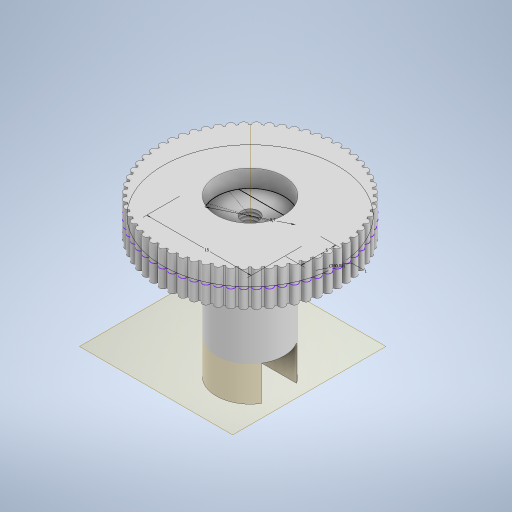
# Autodesk Inventor part: Justage_Knopf
Saved by Autodesk Inventor 2024 (Build 280153000, 153)
## iProperties
Created: 2024-03-07
Part Number: Justage_Knopf
Material: Generisch
Document SubType Name: Modeling
Designer: s1alknau
Density: 1 g/cm^3
Appearance: Vorgabe
Author: s1alknau
Autodesk Inventor part; units mm, degrees
ref_plane "YZ Plane" through (0, 0, 0) normal (1, 0, 0) x (0, 1, 0)
ref_plane "XZ Plane" through (0, 0, 0) normal (0, 1, 0) x (-1, 0, 0)
ref_plane "XY Plane" through (0, 0, 0) normal (0, 0, 1) x (1, 0, 0)
sketch "Skizze1" plane through (0, 0, 0) normal (0, 0, 1) x (1, 0, 0)
  circle A0 centre (0, 0) radius 4.85
  arc A1 (12.49, -0.4999) -> (12.49, 0.4999) centre (12.5, 0) ccw
  arc A2 (12.4738, 0.8084) -> (12.3693, 1.8027) centre (12.4315, 1.3066) ccw
  arc A3 (12.321, 2.1078) -> (12.1131, 3.0858) centre (12.2268, 2.5989) ccw
  arc A4 (12.0332, 3.3842) -> (11.7242, 4.3351) centre (11.8882, 3.8627) ccw
  arc A5 (11.6135, 4.6235) -> (11.2069, 5.5368) centre (11.4193, 5.0842) ccw
  arc A6 (11.0666, 5.8121) -> (10.5667, 6.6779) centre (10.8253, 6.25) ccw
  arc A7 (10.3985, 6.937) -> (9.8108, 7.7459) centre (10.1127, 7.3473) ccw
  arc A8 (9.6164, 7.9859) -> (8.9474, 8.7289) centre (9.2893, 8.3641) ccw
  arc A9 (8.7289, 8.9474) -> (7.9859, 9.6164) centre (8.3641, 9.2893) ccw
  arc A10 (7.7459, 9.8108) -> (6.937, 10.3985) centre (7.3473, 10.1127) ccw
  arc A11 (6.6779, 10.5667) -> (5.8121, 11.0666) centre (6.25, 10.8253) ccw
  arc A12 (5.5368, 11.2069) -> (4.6235, 11.6135) centre (5.0842, 11.4193) ccw
  arc A13 (4.3351, 11.7242) -> (3.3842, 12.0332) centre (3.8627, 11.8882) ccw
  arc A14 (3.0858, 12.1131) -> (2.1078, 12.321) centre (2.5989, 12.2268) ccw
  arc A15 (1.8027, 12.3693) -> (0.8084, 12.4738) centre (1.3066, 12.4315) ccw
  arc A16 (0.4999, 12.49) -> (-0.4999, 12.49) centre (0, 12.5) ccw
  arc A17 (-0.8084, 12.4738) -> (-1.8027, 12.3693) centre (-1.3066, 12.4315) ccw
  arc A18 (-2.1078, 12.321) -> (-3.0858, 12.1131) centre (-2.5989, 12.2268) ccw
  arc A19 (-3.3842, 12.0332) -> (-4.3351, 11.7242) centre (-3.8627, 11.8882) ccw
  arc A20 (-4.6235, 11.6135) -> (-5.5368, 11.2069) centre (-5.0842, 11.4193) ccw
  arc A21 (-5.8121, 11.0666) -> (-6.6779, 10.5667) centre (-6.25, 10.8253) ccw
  arc A22 (-6.937, 10.3985) -> (-7.7459, 9.8108) centre (-7.3473, 10.1127) ccw
  arc A23 (-7.9859, 9.6164) -> (-8.7289, 8.9474) centre (-8.3641, 9.2893) ccw
  arc A24 (-8.9474, 8.7289) -> (-9.6164, 7.9859) centre (-9.2893, 8.3641) ccw
  arc A25 (-9.8108, 7.7459) -> (-10.3985, 6.937) centre (-10.1127, 7.3473) ccw
  arc A26 (-10.5667, 6.6779) -> (-11.0666, 5.8121) centre (-10.8253, 6.25) ccw
  arc A27 (-11.2069, 5.5368) -> (-11.6135, 4.6235) centre (-11.4193, 5.0842) ccw
  arc A28 (-11.7242, 4.3351) -> (-12.0332, 3.3842) centre (-11.8882, 3.8627) ccw
  arc A29 (-12.1131, 3.0858) -> (-12.321, 2.1078) centre (-12.2268, 2.5989) ccw
  arc A30 (-12.3693, 1.8027) -> (-12.4738, 0.8084) centre (-12.4315, 1.3066) ccw
  arc A31 (-12.49, 0.4999) -> (-12.49, -0.4999) centre (-12.5, 0) ccw
  arc A32 (-12.4738, -0.8084) -> (-12.3693, -1.8027) centre (-12.4315, -1.3066) ccw
  arc A33 (-12.321, -2.1078) -> (-12.1131, -3.0858) centre (-12.2268, -2.5989) ccw
  arc A34 (-12.0332, -3.3842) -> (-11.7242, -4.3351) centre (-11.8882, -3.8627) ccw
  arc A35 (-11.6135, -4.6235) -> (-11.2069, -5.5368) centre (-11.4193, -5.0842) ccw
  arc A36 (-11.0666, -5.8121) -> (-10.5667, -6.6779) centre (-10.8253, -6.25) ccw
  arc A37 (-10.3985, -6.937) -> (-9.8108, -7.7459) centre (-10.1127, -7.3473) ccw
  arc A38 (-9.6164, -7.9859) -> (-8.9474, -8.7289) centre (-9.2893, -8.3641) ccw
  arc A39 (-8.7289, -8.9474) -> (-7.9859, -9.6164) centre (-8.3641, -9.2893) ccw
  arc A40 (-7.7459, -9.8108) -> (-6.937, -10.3985) centre (-7.3473, -10.1127) ccw
  arc A41 (-6.6779, -10.5667) -> (-5.8121, -11.0666) centre (-6.25, -10.8253) ccw
  arc A42 (-5.5368, -11.2069) -> (-4.6235, -11.6135) centre (-5.0842, -11.4193) ccw
  arc A43 (-4.3351, -11.7242) -> (-3.3842, -12.0332) centre (-3.8627, -11.8882) ccw
  arc A44 (-3.0858, -12.1131) -> (-2.1078, -12.321) centre (-2.5989, -12.2268) ccw
  arc A45 (-1.8027, -12.3693) -> (-0.8084, -12.4738) centre (-1.3066, -12.4315) ccw
  arc A46 (-0.4999, -12.49) -> (0.4999, -12.49) centre (0, -12.5) ccw
  arc A47 (0.8084, -12.4738) -> (1.8027, -12.3693) centre (1.3066, -12.4315) ccw
  arc A48 (2.1078, -12.321) -> (3.0858, -12.1131) centre (2.5989, -12.2268) ccw
  arc A49 (3.3842, -12.0332) -> (4.3351, -11.7242) centre (3.8627, -11.8882) ccw
  arc A50 (4.6235, -11.6135) -> (5.5368, -11.2069) centre (5.0842, -11.4193) ccw
  arc A51 (5.8121, -11.0666) -> (6.6779, -10.5667) centre (6.25, -10.8253) ccw
  arc A52 (6.937, -10.3985) -> (7.7459, -9.8108) centre (7.3473, -10.1127) ccw
  arc A53 (7.9859, -9.6164) -> (8.7289, -8.9474) centre (8.3641, -9.2893) ccw
  arc A54 (8.9474, -8.7289) -> (9.6164, -7.9859) centre (9.2893, -8.3641) ccw
  arc A55 (9.8108, -7.7459) -> (10.3985, -6.937) centre (10.1127, -7.3473) ccw
  arc A56 (10.5667, -6.6779) -> (11.0666, -5.8121) centre (10.8253, -6.25) ccw
  arc A57 (11.2069, -5.5368) -> (11.6135, -4.6235) centre (11.4193, -5.0842) ccw
  arc A58 (11.7242, -4.3351) -> (12.0332, -3.3842) centre (11.8882, -3.8627) ccw
  arc A59 (12.1131, -3.0858) -> (12.321, -2.1078) centre (12.2268, -2.5989) ccw
  arc A60 (12.3693, -1.8027) -> (12.4738, -0.8084) centre (12.4315, -1.3066) ccw
  arc A61 (12.4738, -0.8084) -> (12.49, -0.4999) centre (0, 0) ccw
  arc A62 (12.321, -2.1078) -> (12.3693, -1.8027) centre (0, 0) ccw
  arc A63 (12.0332, -3.3842) -> (12.1131, -3.0858) centre (0, 0) ccw
  arc A64 (11.6135, -4.6235) -> (11.7242, -4.3351) centre (0, 0) ccw
  arc A65 (11.0666, -5.8121) -> (11.2069, -5.5368) centre (0, 0) ccw
  arc A66 (10.3985, -6.937) -> (10.5667, -6.6779) centre (0, 0) ccw
  arc A67 (9.6164, -7.9859) -> (9.8108, -7.7459) centre (0, 0) ccw
  arc A68 (8.7289, -8.9474) -> (8.9474, -8.7289) centre (0, 0) ccw
  arc A69 (7.7459, -9.8108) -> (7.9859, -9.6164) centre (0, 0) ccw
  arc A70 (6.6779, -10.5667) -> (6.937, -10.3985) centre (0, 0) ccw
  arc A71 (5.5368, -11.2069) -> (5.8121, -11.0666) centre (0, 0) ccw
  arc A72 (4.3351, -11.7242) -> (4.6235, -11.6135) centre (0, 0) ccw
  arc A73 (3.0858, -12.1131) -> (3.3842, -12.0332) centre (0, 0) ccw
  arc A74 (1.8027, -12.3693) -> (2.1078, -12.321) centre (0, 0) ccw
  arc A75 (0.4999, -12.49) -> (0.8084, -12.4738) centre (0, 0) ccw
  arc A76 (-0.8084, -12.4738) -> (-0.4999, -12.49) centre (0, 0) ccw
  arc A77 (-2.1078, -12.321) -> (-1.8027, -12.3693) centre (0, 0) ccw
  arc A78 (-3.3842, -12.0332) -> (-3.0858, -12.1131) centre (0, 0) ccw
  arc A79 (-4.6235, -11.6135) -> (-4.3351, -11.7242) centre (0, 0) ccw
  arc A80 (-5.8121, -11.0666) -> (-5.5368, -11.2069) centre (0, 0) ccw
  arc A81 (-6.937, -10.3985) -> (-6.6779, -10.5667) centre (0, 0) ccw
  arc A82 (-7.9859, -9.6164) -> (-7.7459, -9.8108) centre (0, 0) ccw
  arc A83 (-8.9474, -8.7289) -> (-8.7289, -8.9474) centre (0, 0) ccw
  arc A84 (-9.8108, -7.7459) -> (-9.6164, -7.9859) centre (0, 0) ccw
  arc A85 (-10.5667, -6.6779) -> (-10.3985, -6.937) centre (0, 0) ccw
  arc A86 (-11.2069, -5.5368) -> (-11.0666, -5.8121) centre (0, 0) ccw
  arc A87 (-11.7242, -4.3351) -> (-11.6135, -4.6235) centre (0, 0) ccw
  arc A88 (-12.1131, -3.0858) -> (-12.0332, -3.3842) centre (0, 0) ccw
  arc A89 (-12.3693, -1.8027) -> (-12.321, -2.1078) centre (0, 0) ccw
  arc A90 (-12.49, -0.4999) -> (-12.4738, -0.8084) centre (0, 0) ccw
  arc A91 (-12.4738, 0.8084) -> (-12.49, 0.4999) centre (0, 0) ccw
  arc A92 (-12.321, 2.1078) -> (-12.3693, 1.8027) centre (0, 0) ccw
  arc A93 (-12.0332, 3.3842) -> (-12.1131, 3.0858) centre (0, 0) ccw
  arc A94 (-11.6135, 4.6235) -> (-11.7242, 4.3351) centre (0, 0) ccw
  arc A95 (-11.0666, 5.8121) -> (-11.2069, 5.5368) centre (0, 0) ccw
  arc A96 (-10.3985, 6.937) -> (-10.5667, 6.6779) centre (0, 0) ccw
  arc A97 (-9.6164, 7.9859) -> (-9.8108, 7.7459) centre (0, 0) ccw
  arc A98 (-8.7289, 8.9474) -> (-8.9474, 8.7289) centre (0, 0) ccw
  arc A99 (-7.7459, 9.8108) -> (-7.9859, 9.6164) centre (0, 0) ccw
  arc A100 (-6.6779, 10.5667) -> (-6.937, 10.3985) centre (0, 0) ccw
  arc A101 (-5.5368, 11.2069) -> (-5.8121, 11.0666) centre (0, 0) ccw
  arc A102 (-4.3351, 11.7242) -> (-4.6235, 11.6135) centre (0, 0) ccw
  arc A103 (-3.0858, 12.1131) -> (-3.3842, 12.0332) centre (0, 0) ccw
  arc A104 (-1.8027, 12.3693) -> (-2.1078, 12.321) centre (0, 0) ccw
  arc A105 (-0.4999, 12.49) -> (-0.8084, 12.4738) centre (0, 0) ccw
  arc A106 (0.8084, 12.4738) -> (0.4999, 12.49) centre (0, 0) ccw
  arc A107 (2.1078, 12.321) -> (1.8027, 12.3693) centre (0, 0) ccw
  arc A108 (3.3842, 12.0332) -> (3.0858, 12.1131) centre (0, 0) ccw
  arc A109 (4.6235, 11.6135) -> (4.3351, 11.7242) centre (0, 0) ccw
  arc A110 (5.8121, 11.0666) -> (5.5368, 11.2069) centre (0, 0) ccw
  arc A111 (6.937, 10.3985) -> (6.6779, 10.5667) centre (0, 0) ccw
  arc A112 (7.9859, 9.6164) -> (7.7459, 9.8108) centre (0, 0) ccw
  arc A113 (8.9474, 8.7289) -> (8.7289, 8.9474) centre (0, 0) ccw
  arc A114 (9.8108, 7.7459) -> (9.6164, 7.9859) centre (0, 0) ccw
  arc A115 (10.5667, 6.6779) -> (10.3985, 6.937) centre (0, 0) ccw
  arc A116 (11.2069, 5.5368) -> (11.0666, 5.8121) centre (0, 0) ccw
  arc A117 (11.7242, 4.3351) -> (11.6135, 4.6235) centre (0, 0) ccw
  arc A118 (12.1131, 3.0858) -> (12.0332, 3.3842) centre (0, 0) ccw
  arc A119 (12.49, 0.4999) -> (12.4738, 0.8084) centre (0, 0) ccw
  arc A120 (12.3693, 1.8027) -> (12.321, 2.1078) centre (0, 0) ccw
  line L0 (7.5, -2.5) -> (-7.5, -2.5)
  line L1 (-7.5, -2.5) -> (-7.5, 2.5)
  line L2 (-7.5, 2.5) -> (7.5, 2.5)
  line L3 (7.5, 2.5) -> (7.5, -2.5)
  line L4 (7.5, -2.5) -> (-7.5, 2.5) construction
  line L5 (-7.5, -2.5) -> (7.5, 2.5) construction
  point P0 (7.5, 0)
  dimension "d1" = 9.7
  dimension "d3" = 1
  dimension "d6" = 360
  dimension "d19" = 5
  dimension "d20" = 15
  constraints: 120 point on circle, 61 centre point, 12 end point, 3 midpoint, 2 parallel, 1 horizontal, 1 perpendicular, 423 other
  measures "d1" diameter of A0
  measures "d3" diameter of A1
  measures "d19" distance between parallel lines of L2 L0
  measures "d20" distance from line of point (7.5, 0) L1
extrude "Extrusion1" add sketch "Skizze1" along normal mid plane 5 contours A0 L2 L3 L0 | A0 L0 L1 L2 | A61 A60 A62 A59 A63 A58 A64 A57 A65 A56 A66 A55 A67 A54 A68 A53 A69 A52 A70 A51 A71 A50 A72 A49 A73 A48 A74 A47 A75 A46 A76 A45 A77 A44 A78 A43 A79 A42 A80 A41 A81 A40 A82 A39 A83 A38 A84 A37 A85 A36 A86 A35 A87 A34 A88 A33 A89 A32 A90 A31 A91 A30 A92 A29 A93 A28 A94 A27 A95 A26 A96 A25 A97 A24 A98 A23 A99 A22 A100 A21 A101 A20 A102 A19 A103 A18 A104 A17 A105 A16 A106 A15 A107 A14 A108 A13 A109 A12 A110 A11 A111 A10 A112 A9 A113 A8 A114 A7 A115 A6 A116 A5 A117 A4 A118 A3 A120 A2 A119 A1
extrude "Extrusion2" add sketch "Skizze1" against normal blind 20 contours A0 L0 L2 | L2 A0 | A0 L0
extrude "Extrusion3" cut sketch "Skizze1" along normal blind 5 from surface at -20 contours A0 L0 L2 | A0 L2 L3 L0 | A0 L0 L1 L2
ref_plane "Arbeitsebene2" through (0, -2.5, -15) normal (0, 0, 1) x (1, 0, 0)
hole "Bohrung3" at (0, 0, 0) direction (0, 0, -1) diameter 2.459 end through all thread size "M3x0.5" class "6H" standard "ISO Metric profile"
